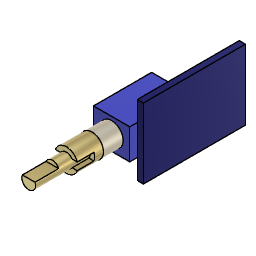
PropWashSim Dual Encoder (6mm screw, 6.5 loose) v4 (Autodesk Fusion 360 design; units mm, degrees)
Autodesk Fusion 360 part; units mm, degrees
sketch "Profile" plane through (0, 0, 0) normal (0, 1, 0) x (1, 0, 0)
  line L0 (4.6, 3.85) -> (-4.6, 3.85)
  line L1 (-4.6, 3.85) -> (-4.6, -3.85)
  line L2 (-4.6, -3.85) -> (4.6, -3.85)
  line L3 (4.6, -3.85) -> (4.6, 3.85)
  line L4 (4.6, 3.85) -> (-4.6, -3.85) construction
  line L5 (-4.6, 3.85) -> (4.6, -3.85) construction
  circle A0 centre (0, 0) radius 2.925
  line L6 (2.235, -1.8869) -> (2.235, 1.8869)
  line L7 (0, 0) -> (0, 6.159) construction
  line L8 (-2.235, -1.8869) -> (-2.235, 1.8869)
  line L9 (-2.7664, -0.95) -> (2.7664, -0.95)
  line L10 (0, 0) -> (1.3963, 0) construction
  line L11 (-2.7664, 0.95) -> (2.7664, 0.95)
  dimension "d1" = 9.2
  dimension "d2" = 7.7
  dimension "d3" = 5.85
  dimension "d17" = 2.235
  dimension "d18" = 0.95
  constraint horizontal L0
  constraint perpendicular L0 L1
  constraint parallel L0 L2
  constraint parallel L1 L3
  constraint coincident L4 A0.centre
  constraint coincident L5 A0.centre
  constraint coincident A0.centre L7.start
  constraint coincident A0 L6.start
  constraint vertical L6
  constraint coincident A0 L6.end
  constraint vertical L7
  constraint symmetric L6.start L7 L8.start
  constraint symmetric L6.end L7 L8.end
  constraint coincident A0 L9.start
  constraint coincident A0 L9.end
  constraint horizontal L9
  constraint perpendicular L7 L10
  constraint symmetric L9.start L10 L11.start
  constraint symmetric L9.end L10 L11.end
  measures "d1" distance of L1.end L2.end
  measures "d2" distance of L0.end L1.end
  measures "d3" diameter of A0
  measures "d17" distance of A0.centre L6
  measures "d18" distance of A0.centre L9
extrude "Extrude1" add sketch "Profile" along normal blind 14.75 contours L0 L1 L2 L3 | A0 L6 L9 L11 | A0 L6 L11 | A0 L6 L9 | A0 L6 L8 L11 | L6 L8 L9 L11 | A0 L6 L8 L9 | A0 L8 L11 | A0 L8 L9 L11 | A0 L8 L9 makes body 1
extrude "Extrude2" add sketch "Profile" against normal blind 5 contours A0 L6 L9 L11 | A0 L6 L11 | A0 L6 L9 | A0 L6 L8 L11 | L6 L8 L9 L11 | A0 L6 L8 L9 | A0 L8 L11 | A0 L8 L9 L11 | A0 L8 L9 bodies 1
extrude "Extrude3" add sketch "Profile" against normal blind 6.5 from surface at -5 separate body contours A0 L6 L11 | A0 L6 L9 | A0 L6 L8 L11 | A0 L6 L8 L9 | A0 L8 L11 | A0 L8 L9 makes body 2 at (1.1749, -9.3333, -2.6787) makes body 3 at (-1.1749, -9.3333, 2.6787)
extrude "Extrude5" add sketch "Profile" against normal blind 2.25 from surface at -5 separate body contours A0 L6 L9 L11 | L6 L8 L9 L11 | A0 L8 L9 L11 makes body 4
combine "Combine1" operation add target body 3 tool bodies 4 2
cylinder "CylinderPrimitive1" add diameter 3.5 height 9.55 placed x (1, 0, 0) y (0, 0, 1) z (0, -1, 0) at (0, -11.5, 0) bodies 3
sketch "PCB" plane through (4.6, 0, 0) normal (1, 0, 0) x (0, 1, 0)
  line L0 (0, 3.85) -> (0, -3.85)
  line L1 (0, -3.85) -> (14.75, -3.85)
  line L2 (14.75, -3.85) -> (14.75, 3.85)
  line L3 (14.75, 3.85) -> (0, 3.85)
  line L4 (27.8, 8.9) -> (1.9, 8.9)
  line L5 (1.9, 8.9) -> (1.9, -8.9)
  line L6 (1.9, -8.9) -> (27.8, -8.9)
  line L7 (27.8, -8.9) -> (27.8, 8.9)
  line L8 (27.8, 8.9) -> (1.9, -8.9) construction
  line L9 (1.9, 8.9) -> (27.8, -8.9) construction
  point P0 (14.85, 0)
  dimension "d12" = 25.9
  dimension "d13" = 17.8
  dimension "d14" = 1.9
  constraint horizontal L4
  constraint perpendicular L4 L5
  constraint parallel L4 L6
  constraint parallel L5 L7
  constraint coincident L8 P0
  constraint coincident L9 P0
  constraint horizontal origin P0
  measures "d12" distance of L5.end L6.end
  measures "d13" distance of L4.end L5.end
  measures "d14" distance of origin L5
extrude "Extrude4" add sketch "PCB" along normal blind 1.55 separate body contours L1 L2 L3 L4 L5 L6 L7 | L1 L2 L3 L5 makes body 5
extrude "Extrude6" add 1 faces at (-0.4497, -11.5, 0.2434) along direction (0, 1, 0) up to surface (4.25 mm away) on bodies 3 bodies 3
sketch "Sketch4" plane through (0, -21.05, 0) normal (0, -1, 0) x (1, 0, 0)
  circle A0 centre (0, 0) radius 1.75
  line L0 (-1.6039, 0.7) -> (1.6039, 0.7)
  dimension "d25" = 2.45
  constraint coincident A0 L0.start
  constraint coincident A0 L0.end
  constraint horizontal L0
extrude "Extrude7" cut sketch "Sketch4" against normal blind 6 contours A0 L0 picked at (-0.2322, 1.2474) bodies 3
equation "d17 = ( 4.47 / 2 ) * 1 mm"
equation "d18 = ( 1.9 / 2 ) * 1 mm"
